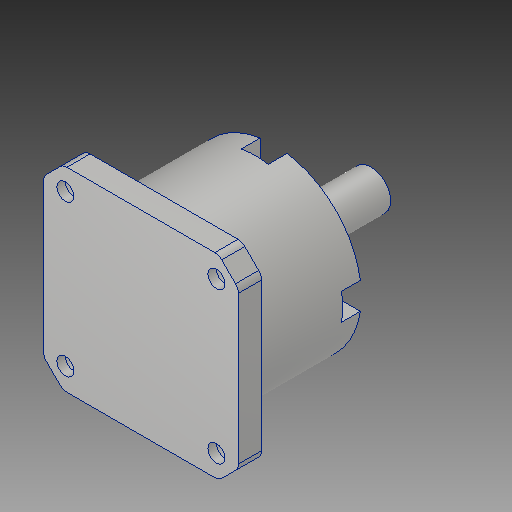
# Autodesk Inventor part: Reducteur
Saved by Autodesk Inventor 2017 (Build 210142000, 142)
## iProperties
Company: FABLAB Frenchmakers
Part Number: Reducteur
Material: ----------
Document SubType Name: Modeling
Designer: FABLAB Frenchmakers
Density: 7.86 g/cm^3
Appearance: Aluminium - Plat
Mass: 243.013 g
Surface Area: 76.4813 cm^2
Volume: 30.9177 cm^3
Project: 1420 Vauban 3D XL
Catalog Web Link: http://frenchmakers.com/
Stock Number: 1420-05-11
Autodesk Inventor part; units mm, degrees
ref_plane "YZ Plane" through (0, 0, 0) normal (1, 0, 0) x (0, 1, 0)
ref_plane "XZ Plane" through (0, 0, 0) normal (0, 1, 0) x (-1, 0, 0)
ref_plane "XY Plane" through (0, 0, 0) normal (0, 0, 1) x (1, 0, 0)
sketch "Esquisse1" plane through (0, 0, 0) normal (0, 0, 1) x (1, 0, 0)
  line L0 (-20, -20) -> (20, -20)
  line L1 (20, -20) -> (20, 20)
  line L2 (20, 20) -> (-20, 20)
  line L3 (-20, 20) -> (-20, -20)
  line L4 (-20, -20) -> (20, 20) construction
  line L5 (20, -20) -> (-20, 20) construction
  point P0 (0, 0)
  dimension "d0" = 40
  dimension "d1" = 40
  constraints: 12 end point, 2 midpoint, 2 parallel, 1 horizontal, 1 perpendicular
  measures "d0" distance between parallel lines of L1 L3
  measures "d1" distance between parallel lines of L0 L2
extrude "Extrusion1" add sketch "Esquisse1" along normal blind 4.75
sketch "Esquisse2" plane through (0, 0, 0) normal (0, 0, -1) x (-1, 0, 0)
  circle A0 centre (0, 0) radius 18
  dimension "d4" = 36
  constraints: 1 centre point, 1 coincident
  measures "d4" diameter of A0
extrude "Extrusion2" add sketch "Esquisse2" along normal blind 22.5
sketch "Esquisse3" plane through (0, 0, -22.5) normal (0, 0, -1) x (-1, 0, 0)
  circle A0 centre (0, 0) radius 11
  dimension "d7" = 22
  constraints: 1 centre point, 1 coincident
  measures "d7" diameter of A0
extrude "Extrusion3" add sketch "Esquisse3" along normal blind 2
sketch "Esquisse4" plane through (0, 0, -24.5) normal (0, 0, -1) x (-1, 0, 0)
  circle A0 centre (0, 0) radius 4
  dimension "d10" = 8
  constraints: 1 centre point, 1 coincident
  measures "d10" diameter of A0
extrude "Extrusion4" add sketch "Esquisse4" along normal blind 18
sketch "Esquisse5" plane through (0, 0, -22.5) normal (0, 0, -1) x (-1, 0, 0)
  line L0 (2.75, 14) -> (2.75, 20)
  line L1 (2.75, 20) -> (-2.75, 20)
  line L2 (-2.75, 20) -> (-2.75, 14)
  arc A0 (-2.75, 14) -> (2.75, 14) centre (0, 14) ccw
  line L3 (-5.8727, 11.25) -> (6.9121, 11.25) construction
  line L4 (-20, 20) -> (20, 20) construction
  point P0 (0, 0)
  dimension "d13" = 5.5
  dimension "d14" = 11.25
  constraints: 8 end point, 3 tangent, 2 point on circle, 1 centre point, 1 collinear, 1 horizontal, 1 parallel, 1 vertical, 1 vertical alignment
  measures "d13" distance between parallel lines of L0 L2
  measures "d14" distance from line of point (0, 0) L3
extrude "Extrusion5" cut sketch "Esquisse5" against normal blind 3.85
pattern_circular "Réseau circulaire1" count 4 over 360 about axis through (0, 0, 0) along (0, 0, -1) of "Extrusion5"
sketch "Esquisse6" plane through (0, 0, -22.5) normal (0, 0, -1) x (-1, 0, 0)
  circle A0 centre (0, 0) radius 14 construction
  circle A1 centre (0, 0) radius 11 construction
  line L0 (0, 0) -> (-20.9292, 20.9292) construction
  line L1 (28, 0) -> (-28, 0) construction
  point P0 (-9.8995, 9.8995)
  dimension "d20" = 28
  dimension "d21" = 45
  constraints: 2 end point, 1 coincident, 1 point on line, 3 other
  measures "d21" angle of L0 L1
hole "Perçage1" at (9.8995, 9.8995, -22.5) direction (0, 0, 1) diameter 2.459 depth 8.8 tip angle 118 thread size "M3x0.5" class "6H" standard "ISO Metric profile"
pattern_circular "Réseau circulaire2" count 4 over 360 about axis through (0, 0, 0) along (0, 0, -1) of "Perçage1"
sketch "Esquisse7" plane through (0, 0, 0) normal (0, 0, -1) x (-1, 0, 0)
  point P0 (0, 0)
  point P1 (15.5, 15.5)
  point P2 (15.5, -15.5)
  point P3 (-15.5, -15.5)
  point P4 (-15.5, 15.5)
  dimension "d32" = 31
  dimension "d33" = 31
  dimension "d34" = 15.5
  dimension "d35" = 15.5
  constraints: 2 horizontal alignment, 2 vertical alignment
  measures "d32" distance of point (15.5, -15.5) point (15.5, 15.5)
  measures "d33" distance of point (-15.5, -15.5) point (15.5, -15.5)
  measures "d34" horizontal distance of point (0, 0) point (15.5, -15.5)
  measures "d35" horizontal distance of point (0, 0) point (15.5, -15.5)
hole "Perçage2" at (-15.5, 15.5, 0) at (-15.5, -15.5, 0) at (15.5, -15.5, 0) at (15.5, 15.5, 0) direction (0, 0, 1) diameter 3.5 end through all counterbore diameter 6 counterbore depth 3
chamfer "Chanfrein1" distance 4 angle 45 4 edges at (-20, -20, 2.375) (20, -20, 2.375) (20, 20, 2.375) (-20, 20, 2.375)
fillet "Congé1" radius 2 8 edges at (-16, -20, 2.375) (16, -20, 2.375) (20, -16, 2.375) (20, 16, 2.375) (16, 20, 2.375) (-16, 20, 2.375) (-20, 16, 2.375) (-20, -16, 2.375)
equation "\"d33\" = d32"
equation "\"d34\" = 0.5 * d32"
equation "\"d35\" = 0.5 * d33"
